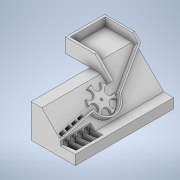
# Autodesk Inventor part: github
Saved by Autodesk Inventor 2020 (Build 240168000, 168)
## iProperties
Created: 2020-12-24
Part Number: github
Material: 一般
Document SubType Name: Modeling
Designer: Sugar
Density: 1 g/cm^3
Appearance: 預設
Author: Sugar
Autodesk Inventor part; units mm, degrees
ref_plane "YZ Plane" through (0, 0, 0) normal (1, 0, 0) x (0, 1, 0)
ref_plane "XZ Plane" through (0, 0, 0) normal (0, 1, 0) x (-1, 0, 0)
ref_plane "XY Plane" through (0, 0, 0) normal (0, 0, 1) x (1, 0, 0)
sketch "草圖2" plane through (0, 0, 0) normal (1, 0, 0) x (0, 1, 0)
  line L0 (0, 0) -> (300, 0)
  line L1 (300, 0) -> (300, 150)
  line L2 (300, 150) -> (150, 300)
  line L3 (150, 300) -> (100, 300)
  line L4 (100, 300) -> (100, 450)
  line L5 (100, 450) -> (0, 450)
  line L6 (0, 450) -> (0, 0)
  dimension "d0" = 300
  dimension "d1" = 450
  dimension "d2" = 150
  dimension "d3" = 150
  dimension "d4" = 100
  dimension "d5" = 50
  constraints: 14 end point, 4 perpendicular, 1 horizontal, 1 parallel
  measures "d0" distance of L0.start L0.end
  measures "d1" distance of L5.end L0.start
  measures "d2" distance of L0.end L1.end
  measures "d3" horizontal distance of L1.end L2.end
  measures "d4" distance of L4.end L5.end
  measures "d5" distance of L2.end L3.end
extrude "擠出1" add sketch "草圖2" along normal blind 600
sketch "草圖3" plane through (0, 150, 300) normal (0, 0.7071068, 0.7071068) x (1, 0, 0)
  line L0 (0, -212.132) -> (0, 106.066) projected
  line L1 (0, 0) -> (600, 0) projected
  line L2 (600, 106.066) -> (600, 318.1981) projected
  line L3 (0, 0) -> (350, 61.8718)
  line L4 (600, 106.066) -> (600, 121.066)
  line L5 (350, 76.8718) -> (0, 15)
  line L6 (0, 15) -> (0, 0)
  line L7 (350, 76.8718) -> (350, 61.8718)
  line L8 (600, 212.132) -> (600, 0) projected
  dimension "d11" = 15
  dimension "d31" = 250
  dimension "d32" = 15
  dimension "d33" = 14.771
  constraints: 10 end point, 2 parallel, 2 point on line, 1 collinear, 1 vertical
  measures "d11" distance of L2.start L4.end
  measures "d31" distance between parallel lines of L2 L7
  measures "d32" distance of L5.start L3.end
  measures "d33" distance between parallel lines of L3 L5
extrude "擠出3" add sketch "草圖3" along normal blind 60
sketch "草圖4" plane through (0, 300, 150) normal (0, 0.7071068, 0.7071068) x (1, 0, 0)
  circle A0 centre (225.2442, -146.9052) radius 10.25 construction
  circle A1 centre (179.5282, -153.9712) radius 11.25 construction
  circle A2 centre (98.546, -166.256) radius 13.25 construction
  circle A3 centre (46.5483, -174.4324) radius 14.25 construction
  line L0 (8.637, -195.6052) -> (251.57, -152.6603) construction
  line L1 (0, -197.132) -> (350, -135.2602) construction
  line L2 (14.7334, -165.5856) -> (63.97, -156.8817)
  line L3 (63.97, -156.8817) -> (68.9312, -184.9466)
  line L4 (14.7334, -165.5856) -> (19.6946, -193.6505)
  line L5 (88.6259, -181.465) -> (84.0128, -155.3696)
  line L6 (84.0128, -155.3696) -> (133.2494, -146.6658)
  line L7 (133.2494, -146.6658) -> (137.8625, -172.7612)
  line L8 (157.5571, -169.2796) -> (153.6404, -147.1231)
  line L9 (153.6404, -147.1231) -> (202.877, -138.4193)
  line L10 (202.877, -138.4193) -> (206.7937, -160.5757)
  line L11 (226.4883, -157.0942) -> (222.9198, -136.9072)
  line L12 (222.9198, -136.9072) -> (272.1563, -128.2033)
  line L13 (272.1563, -128.2033) -> (275.7249, -148.3903)
  line L14 (19.6946, -193.6505) -> (68.9312, -184.9466)
  line L15 (88.6259, -181.465) -> (137.8625, -172.7612)
  line L16 (157.5571, -169.2796) -> (206.7937, -160.5757)
  line L17 (226.4883, -157.0942) -> (275.7249, -148.3903)
  point P0 (0, -106.066)
  point P1 (600, -91.066)
  dimension "d17" = 20.5
  dimension "d18" = 22.5
  dimension "d19" = 26.5
  dimension "d20" = 28.5
  dimension "d21" = 50
  dimension "d22" = 50
  dimension "d23" = 50
  dimension "d24" = 50
  dimension "d25" = 20
  dimension "d26" = 20
  dimension "d27" = 20
  dimension "d28" = 20
  constraints: 34 end point, 10 perpendicular, 8 tangent, 4 centre point, 3 point on line, 2 collinear, 12 other
  measures "d17" diameter of A0
  measures "d18" diameter of A1
  measures "d19" diameter of A2
  measures "d20" diameter of A3
  measures "d21" distance between parallel lines of L4 L3
  measures "d22" distance between parallel lines of L7 L5
  measures "d23" distance between parallel lines of L10 L8
  measures "d24" distance between parallel lines of L13 L11
  measures "d25" distance between parallel lines of L10 L11
  measures "d26" distance between parallel lines of L7 L8
  measures "d27" distance between parallel lines of L3 L5
  measures "d28" distance from line of point (0, -197.132) L4
extrude "擠出4" cut sketch "草圖4" against normal blind 60
sketch "草圖5" plane through (350, 246.783, 288.0698) normal (-0.1740777, 0.6963106, -0.6963106) x (-0.9847319, -0.1230915, 0.1230915)
  line L0 (2.6112, -60) -> (358.0378, -60) projected
  line L1 (-8.4274, -60) -> (-8.4274, -120)
  line L2 (358.0378, -60) -> (2.6112, -60)
  line L3 (359.7659, -70) -> (-2.5175, -70)
  line L4 (125.4267, -120) -> (75.4267, -120) projected
  line L5 (75.4267, -120) -> (125.4267, -120) projected
  line L6 (195.4267, -120) -> (145.4267, -120) projected
  line L7 (145.4267, -120) -> (195.4267, -120) projected
  line L8 (265.4267, -120) -> (215.4267, -120) projected
  line L9 (215.4267, -120) -> (265.4267, -120) projected
  line L10 (335.4267, -120) -> (285.4267, -120) projected
  line L11 (285.4267, -120) -> (335.4267, -120) projected
  line L12 (75.4267, -120) -> (75.4267, -70)
  line L13 (75.4267, -120) -> (125.4267, -120)
  line L14 (125.4267, -120) -> (125.4267, -70)
  line L15 (145.4267, -70) -> (145.4267, -120)
  line L16 (145.4267, -120) -> (195.4267, -120)
  line L17 (195.4267, -120) -> (195.4267, -70)
  line L18 (215.4267, -70) -> (215.4267, -120)
  line L19 (215.4267, -120) -> (265.4267, -120)
  line L20 (265.4267, -120) -> (265.4267, -70)
  line L21 (285.4267, -70) -> (285.4267, -120)
  line L22 (285.4267, -120) -> (335.4267, -120)
  line L23 (335.4267, -120) -> (335.4267, -70)
  point P0 (339.5741, -378.1981)
  point P1 (75.4267, -120)
  point P2 (195.4267, -120)
  point P3 (215.4267, -120)
  point P4 (335.4267, -120)
  point P5 (285.4267, -120)
  dimension "d34" = 60
  dimension "d35" = 10
  constraints: 28 end point, 5 perpendicular, 3 horizontal, 3 parallel, 3 vertical, 1 collinear, 1 point on line, 11 other
  measures "d34" distance of L1.start L1.end
extrude "擠出7" cut sketch "草圖5" against normal blind 126 contours L14 L4 L12 L3
extrude "擠出8" cut sketch "草圖5" against normal blind 115 contours L17 L6 L15 L3
extrude "擠出9" cut sketch "草圖5" against normal blind 110 contours L20 L8 L18 L3
extrude "擠出10" cut sketch "草圖5" against normal blind 95 contours L23 L10 L21 L3
sketch "草圖10" plane through (0, 100, 450) normal (0, 1, 0) x (1, 0, 0)
  line L0 (33.694, 114.1421) -> (29.2117, 150) projected
  line L1 (79.987, 150) -> (84.4692, 114.1421) projected
  line L2 (104.7793, 114.1421) -> (100.2971, 150) projected
  line L3 (151.0723, 150) -> (155.5546, 114.1421) projected
  line L4 (175.8647, 114.1421) -> (171.3824, 150) projected
  line L5 (222.1577, 150) -> (226.6399, 114.1421) projected
  line L6 (246.5073, 117.6838) -> (242.4678, 150) projected
  line L7 (293.243, 150) -> (295.7439, 129.993) projected
  line L8 (0, 150) -> (600, 150) projected
  line L9 (24.1728, 150) -> (39.1728, 30)
  line L10 (39.1728, 30) -> (100.0259, 30)
  line L11 (100.0259, 30) -> (85.0259, 150)
  line L12 (24.1728, 150) -> (85.0259, 150)
  line L13 (95.2582, 150) -> (110.2582, 30)
  line L14 (110.2582, 30) -> (171.1112, 30)
  line L15 (171.1112, 30) -> (156.1112, 150)
  line L16 (95.2582, 150) -> (156.1112, 150)
  line L17 (166.3435, 150) -> (181.3435, 30)
  line L18 (181.3435, 30) -> (242.1966, 30)
  line L19 (242.1966, 30) -> (227.1966, 150)
  line L20 (166.3435, 150) -> (227.1966, 150)
  line L21 (237.4288, 150) -> (252.4288, 30)
  line L22 (252.4288, 30) -> (313.2819, 30)
  line L23 (313.2819, 30) -> (298.2819, 150)
  line L24 (237.4288, 150) -> (298.2819, 150)
  line L25 (0, 0) -> (600, 0) projected
  point P0 (0, 450)
  point P1 (225.9422, 119.7233)
  point P2 (294.8735, 136.9561)
  point P3 (245.6369, 124.647)
  point P4 (225.9422, 119.7233)
  point P5 (104.7793, 114.1421)
  point P6 (155.5546, 114.1421)
  point P7 (33.694, 114.1421)
  point P8 (84.4692, 114.1421)
  point P9 (24.1728, 150)
  dimension "d17" = 20.5
  dimension "d18" = 22.5
  dimension "d19" = 26.5
  dimension "d20" = 28.5
  dimension "d21" = 50
  dimension "d22" = 50
  dimension "d23" = 50
  dimension "d24" = 50
  dimension "d25" = 20
  dimension "d26" = 20
  dimension "d27" = 20
  dimension "d28" = 20
  dimension "d39" = 30
  dimension "d40" = 30
  dimension "d41" = 30
  dimension "d42" = 30
  dimension "d45" = 5
  dimension "d46" = 5
  dimension "d47" = 5
  dimension "d48" = 5
  dimension "d49" = 5
  dimension "d50" = 5
  dimension "d51" = 5
  dimension "d52" = 5
  constraints: 32 end point, 13 parallel, 4 point on line
  measures "d39" distance between parallel lines of L25 L10
  measures "d40" distance between parallel lines of L25 L14
  measures "d41" distance between parallel lines of L25 L18
  measures "d42" distance between parallel lines of L25 L22
  measures "d45" distance between parallel lines of L11 L1
  measures "d46" distance between parallel lines of L0 L9
  measures "d47" distance between parallel lines of L2 L13
  measures "d48" distance between parallel lines of L15 L3
  measures "d49" distance between parallel lines of L4 L17
  measures "d50" distance between parallel lines of L5 L19
  measures "d51" distance between parallel lines of L7 L23
  measures "d52" distance between parallel lines of L6 L21
extrude "擠出6" cut sketch "草圖10" against normal blind 65
sketch "草圖11" plane through (0, 300, 150) normal (0, 0.7071068, 0.7071068) x (1, 0, 0)
  circle A0 centre (477.6204, -106.066) radius 127.6204
  line L0 (600, 0) -> (600, -212.132) projected
  line L1 (350, -135.2602) -> (350, -150.2602) projected
  point P0 (0, -106.066)
  point P1 (600, -106.066)
  point P2 (600, -142.2624)
  point P3 (600, -69.8697)
  constraints: 1 centre point, 1 horizontal alignment, 1 midpoint, 1 tangent
extrude "擠出11" add sketch "草圖11" along normal blind 20
sketch "草圖12" plane through (0, 314.1421, 164.1421) normal (0, 0.7071068, 0.7071068) x (1, 0, 0)
  circle A0 centre (477.6204, -106.066) radius 127.6204 projected
  circle A1 centre (477.6204, -106.066) radius 10
  circle A2 centre (402.5525, -36.0873) radius 40
  line L0 (0, -106.066) -> (600, -106.066) projected
  circle A3 centre (379.4831, -136.0873) radius 40
  circle A4 centre (454.551, -206.066) radius 40
  circle A5 centre (552.6882, -176.0447) radius 40
  circle A6 centre (575.7576, -76.0447) radius 40
  circle A7 centre (500.6897, -6.066) radius 40
  line L1 (500.6897, -6.066) -> (477.6204, -106.066) construction
  line L2 (364.1482, -99.1436) -> (350.0043, -105.0145)
  line L3 (394.818, -173.0311) -> (374.6185, -181.4157)
  line L4 (364.1482, -99.1436) -> (394.818, -173.0311) construction
  line L5 (415.5747, -197.0744) -> (493.5272, -215.0576) construction
  line L6 (454.551, -206.066) -> (477.6204, -106.066) construction
  line L7 (415.5747, -197.0744) -> (411.4018, -215.1626)
  line L8 (493.5272, -215.0576) -> (489.3544, -233.1458)
  line L9 (552.6882, -176.0447) -> (477.6204, -106.066) construction
  line L10 (525.4131, -205.3034) -> (579.9633, -146.786) construction
  line L11 (402.5525, -36.0873) -> (477.6204, -106.066) construction
  line L12 (379.4831, -136.0873) -> (477.6204, -106.066) construction
  line L13 (575.7576, -76.0447) -> (477.6204, -106.066) construction
  line L14 (525.4131, -205.3034) -> (538.9915, -217.9612)
  line L15 (579.9633, -146.786) -> (593.5417, -159.4439)
  line L16 (564.0564, -37.7944) -> (587.4588, -114.295) construction
  line L17 (564.0564, -37.7944) -> (581.8076, -32.3641)
  line L18 (587.4588, -114.295) -> (605.21, -108.8647)
  line L19 (461.7135, 2.9256) -> (465.8863, 21.0137)
  line L20 (500.6897, -6.066) -> (539.666, -15.0576) construction
  line L21 (500.6897, -6.066) -> (461.7135, 2.9256) construction
  line L22 (539.666, -15.0576) -> (543.8389, 3.0306)
  line L23 (375.2774, -65.346) -> (429.8276, -6.8287) construction
  line L24 (375.2774, -65.346) -> (361.699, -52.6881)
  line L25 (429.8276, -6.8287) -> (416.2492, 5.8292)
  point P0 (600, -69.8697)
  point P1 (600, -142.2624)
  point P2 (471.6228, 21.4133)
  point P3 (538.8571, 5.9028)
  point P4 (605.2066, -103.1142)
  point P5 (585.0219, -37.1323)
  point P6 (591.0195, -164.6117)
  point P7 (543.9698, -215.083)
  point P8 (416.3836, -218.0348)
  point P9 (483.6179, -233.5454)
  point P10 (350.0341, -109.0178)
  point P11 (370.2188, -174.9997)
  point P12 (411.2709, 2.951)
  point P13 (364.2212, -47.5203)
  dimension "d63" = 20
  dimension "d64" = 80
  dimension "d67" = 360
  dimension "d69" = 100
  constraints: 50 end point, 17 perpendicular, 17 point on circle, 7 centre point, 5 midpoint, 5 tangent, 1 coincident, 1 collinear, 26 other
  measures "d63" diameter of A1
  measures "d64" diameter of A2
  measures "d69" vertical distance of L1.start L1.end
extrude "擠出12" cut sketch "草圖12" against normal blind 20 contours A0 A6 L17 | L22 A7 A0 | A0 A6 | A7 A0 | A0 L18 A6 | A7 L19 A0 | L0 A1 | A1 L0 | L25 A2 A0 | A0 A5 L15 | A3 A0 L0 | L0 A3 | A2 A0 | A0 A5 | A3 A0 L0 | L0 A0 L2 A3 | A2 L24 A0 | A0 L14 A5 | L3 A0 A3 | A0 A4 L8 | L7 A4 A0 | A0 A4 picked at (578.5347, -74.0136) picked at (502.7839, -3.1882) picked at (399.3169, -34.7769) picked at (556.034, -177.2583) picked at (455.0481, -209.5281)
sketch "草圖13" plane through (0, 314.1421, 164.1421) normal (0, 0.7071068, 0.7071068) x (1, 0, 0)
  arc A0 (394.818, -173.0311) -> (364.1482, -99.1436) centre (379.4831, -136.0873) ccw projected
  arc A1 (593.5417, -159.4439) -> (605.21, -108.8647) centre (477.6204, -106.066) ccw projected
  arc A2 (493.5272, -215.0576) -> (415.5747, -197.0744) centre (454.551, -206.066) ccw projected
  arc A3 (581.8076, -32.3641) -> (543.8389, 3.0306) centre (477.6204, -106.066) ccw projected
  arc A4 (579.9633, -146.786) -> (525.4131, -205.3034) centre (552.6882, -176.0447) ccw projected
  arc A5 (465.8863, 21.0137) -> (416.2492, 5.8292) centre (477.6204, -106.066) ccw projected
  arc A6 (564.0564, -37.7944) -> (587.4588, -114.295) centre (575.7576, -76.0447) ccw projected
  arc A7 (361.699, -52.6881) -> (350.0043, -105.0145) centre (477.6204, -106.066) ccw projected
  arc A8 (461.7135, 2.9256) -> (539.666, -15.0576) centre (500.6897, -6.066) ccw projected
  arc A9 (374.6185, -181.4157) -> (411.4018, -215.1626) centre (477.6204, -106.066) ccw projected
  arc A10 (375.2774, -65.346) -> (429.8276, -6.8287) centre (402.5525, -36.0873) ccw projected
  arc A11 (489.3544, -233.1458) -> (538.9915, -217.9612) centre (477.6204, -106.066) ccw projected
  circle A12 centre (477.6204, -106.066) radius 10 projected
  line L0 (0, -212.132) -> (350, -150.2602) projected
  arc A13 (350, -150.2602) -> (610.3108, -131.2321) centre (477.6204, -106.066) ccw
  arc A14 (335.0608, -152.9011) -> (625.5508, -131.2321) centre (477.6204, -106.066) ccw
  line L1 (350, -135.2602) -> (350, -150.2602) projected
  line L2 (350, -150.2602) -> (335.0608, -152.9011)
  line L3 (610.3108, -131.2321) -> (625.5508, -131.2321)
  line L4 (394.818, -173.0311) -> (374.6185, -181.4157) projected
  line L5 (411.4018, -215.1626) -> (415.5747, -197.0744) projected
  line L6 (493.5272, -215.0576) -> (489.3544, -233.1458) projected
  line L7 (538.9915, -217.9612) -> (525.4131, -205.3034) projected
  line L8 (579.9633, -146.786) -> (593.5417, -159.4439) projected
  line L9 (605.21, -108.8647) -> (587.4588, -114.295) projected
  line L10 (564.0564, -37.7944) -> (581.8076, -32.3641) projected
  line L11 (543.8389, 3.0306) -> (539.666, -15.0576) projected
  line L12 (461.7135, 2.9256) -> (465.8863, 21.0137) projected
  line L13 (416.2492, 5.8292) -> (429.8276, -6.8287) projected
  line L14 (375.2774, -65.346) -> (361.699, -52.6881) projected
  line L15 (350.0043, -105.0145) -> (364.1482, -99.1436) projected
  point P0 (0, -106.066)
  dimension "d72" = 15
  constraints: 5 end point, 4 point on circle, 2 centre point, 2 coincident, 1 horizontal, 1 point on line
  measures "d72" radial gap between concentric circles of A14 A13
extrude "擠出13" add sketch "草圖13" along normal mid plane 80 contours L0 A13 L3 A14
sketch "草圖14" plane through (0, 150, 300) normal (0, 0.7071068, 0.7071068) x (1, 0, 0)
  line L0 (600, -212.132) -> (600, 106.066) projected
  line L1 (600, 8.2369) -> (304.413, 8.2369)
  line L2 (304.413, 8.2369) -> (304.413, -70.0383)
  line L3 (304.413, -70.0383) -> (600, -70.0383)
  line L4 (600, -70.0383) -> (600, 8.2369)
  arc A0 (396.2317, -20) -> (559.009, -20) centre (477.6204, 106.066) ccw projected
  line L5 (298.2819, -35.3553) -> (313.2819, -120.2082) projected
  point P0 (0, 106.066)
  point P1 (600, -70.0383)
  constraints: 8 end point, 2 parallel, 2 point on line, 1 horizontal, 1 perpendicular
extrude "擠出14" add sketch "草圖14" against normal blind 85
sketch "草圖15" plane through (0, 300, 150) normal (0, 0.7071068, 0.7071068) x (1, 0, 0)
  line L0 (600, -106.066) -> (600, 106.066) projected
  line L1 (0, 0) -> (600, 0)
  line L2 (600, 0) -> (600, 56.5167)
  line L3 (600, 56.5167) -> (0, 56.5167)
  line L4 (0, 56.5167) -> (0, 0)
  point P0 (0, -106.066)
  point P1 (600, 0)
  constraints: 8 end point, 2 parallel, 1 horizontal, 1 perpendicular, 1 point on line
extrude "擠出15" add sketch "草圖15" against normal blind 80
sketch "草圖17" plane through (600, 0, 0) normal (1, 0, 0) x (0, 0, -1)
  line L0 (-228.1059, 221.8941) -> (-110.0367, 339.9633) projected
  line L1 (-228.1059, 221.8941) -> (-250.5947, 199.4053) projected
  line L2 (-250.5947, 199.4053) -> (-265.3937, 184.6063) projected
  line L3 (-265.3937, 184.6063) -> (-251.2516, 170.4642) projected
  line L4 (-251.2516, 170.4642) -> (-272.2581, 149.4576) projected
  line L5 (-272.2581, 149.4576) -> (-286.4002, 163.5998) projected
  line L6 (-286.4002, 163.5998) -> (-349.5246, 100.4754) projected
  line L7 (-349.5246, 100.4754) -> (-349.0491, 100) projected
  line L8 (-349.0491, 100) -> (-450, 100) projected
  line L9 (-450, 100) -> (-450, 0) projected
  line L10 (-450, 0) -> (0, 0) projected
  line L11 (0, 0) -> (0, 300) projected
  line L12 (0, 300) -> (-70.0734, 300) projected
  line L13 (-110.0367, 339.9633) -> (-70.0734, 300) projected
  line L14 (0, 300) -> (-70.0734, 300) projected
  line L15 (-450, 0) -> (0, 0) projected
  line L16 (0, 300) -> (-150, 300)
  line L17 (-150, 300) -> (-150, 0)
  line L18 (-150, 0) -> (0, 0)
  line L19 (0, 0) -> (0, 300)
  line L20 (-286.4002, 163.5998) -> (-286.4002, 0)
  line L21 (-150, 300) -> (-286.4002, 163.5998)
  line L22 (-295.1714, 154.8286) -> (-246.1981, 203.8019) projected
  line L23 (-286.4002, 163.5998) -> (-349.5246, 100.4754)
  line L24 (-267.4264, 182.5736) -> (-302.0687, 147.9313) projected
  line L25 (-350, 100) -> (-450, 100)
  line L26 (-450, 100) -> (-450, 0)
  line L27 (-450, 0) -> (-286.4002, 0)
  point P0 (-150, 0)
  point P1 (-70.0734, 300)
  point P2 (-253.7934, 196.2066)
  point P3 (-286.4002, 0)
  point P4 (-289.3527, 160.6473)
  constraints: 20 end point, 4 point on line, 3 collinear, 2 horizontal, 2 parallel, 2 perpendicular, 1 vertical
extrude "擠出16" add sketch "草圖17" along normal blind 400 contours L0 L17 L10 L20 L5 L4 L3 L2 L1 | L16 L12 L11 L10 L17 | L3 L4 L5 L21
sketch "草圖18" plane through (0, 339.9633, 110.0367) normal (0, 0.7071068, 0.7071068) x (1, 0, 0)
  line L0 (600, -56.5167) -> (600, 0) projected
  line L1 (600, 0) -> (0, 0) projected
  line L2 (0, 0) -> (0, -253.6487) projected
  line L3 (0, -253.6487) -> (19.6946, -250.1671) projected
  line L4 (19.6946, -250.1671) -> (14.7334, -222.1023) projected
  line L5 (14.7334, -222.1023) -> (63.97, -213.3984) projected
  line L6 (63.97, -213.3984) -> (68.9312, -241.4633) projected
  line L7 (68.9312, -241.4633) -> (88.6259, -237.9817) projected
  line L8 (88.6259, -237.9817) -> (84.0128, -211.8863) projected
  line L9 (84.0128, -211.8863) -> (133.2494, -203.1824) projected
  line L10 (133.2494, -203.1824) -> (137.8625, -229.2778) projected
  line L11 (137.8625, -229.2778) -> (157.5571, -225.7963) projected
  line L12 (157.5571, -225.7963) -> (153.6404, -203.6398) projected
  line L13 (153.6404, -203.6398) -> (202.877, -194.9359) projected
  line L14 (202.877, -194.9359) -> (206.7937, -217.0924) projected
  line L15 (206.7937, -217.0924) -> (226.4883, -213.6108) projected
  line L16 (226.4883, -213.6108) -> (222.9198, -193.4238) projected
  line L17 (222.9198, -193.4238) -> (272.1563, -184.7199) projected
  line L18 (272.1563, -184.7199) -> (275.7249, -204.907) projected
  line L19 (275.7249, -204.907) -> (350, -191.7769) projected
  line L20 (350, -191.7769) -> (350, -206.7769) projected
  arc A0 (350, -206.7769) -> (610.3108, -187.7487) centre (477.6204, -162.5827) ccw projected
  line L21 (625.5508, -187.7487) -> (610.3108, -187.7487) projected
  arc A1 (600, -249.4157) -> (625.5508, -187.7487) centre (477.6204, -162.5827) ccw projected
  line L22 (600, -249.4157) -> (1000, -249.4157) projected
  line L23 (1000, -56.5167) -> (1000, -249.4157) projected
  line L24 (600, -56.5167) -> (1000, -56.5167) projected
  line L25 (587.4588, -170.8116) -> (605.21, -165.3813) projected
  arc A2 (593.5417, -215.9606) -> (605.21, -165.3813) centre (477.6204, -162.5827) ccw projected
  line L26 (579.9633, -203.3027) -> (593.5417, -215.9606) projected
  arc A3 (579.9633, -203.3027) -> (525.4131, -261.82) centre (552.6882, -232.5614) ccw projected
  line L27 (525.4131, -261.82) -> (538.9915, -274.4779) projected
  arc A4 (489.3544, -289.6624) -> (538.9915, -274.4779) centre (477.6204, -162.5827) ccw projected
  line L28 (489.3544, -289.6624) -> (493.5272, -271.5743) projected
  arc A5 (493.5272, -271.5743) -> (415.5747, -253.5911) centre (454.551, -262.5827) ccw projected
  line L29 (415.5747, -253.5911) -> (411.4018, -271.6792) projected
  arc A6 (374.6185, -237.9323) -> (411.4018, -271.6792) centre (477.6204, -162.5827) ccw projected
  line L30 (394.818, -229.5477) -> (374.6185, -237.9323) projected
  arc A7 (394.818, -229.5477) -> (364.1482, -155.6603) centre (379.4831, -192.604) ccw projected
  line L31 (350.0043, -161.5312) -> (364.1482, -155.6603) projected
  arc A8 (361.699, -109.2048) -> (350.0043, -161.5312) centre (477.6204, -162.5827) ccw projected
  line L32 (375.2774, -121.8627) -> (361.699, -109.2048) projected
  arc A9 (375.2774, -121.8627) -> (429.8276, -63.3453) centre (402.5525, -92.604) ccw projected
  line L33 (429.8276, -63.3453) -> (416.2492, -50.6875) projected
  arc A10 (465.8863, -35.5029) -> (416.2492, -50.6875) centre (477.6204, -162.5827) ccw projected
  line L34 (465.8863, -35.5029) -> (461.7135, -53.5911) projected
  arc A11 (461.7135, -53.5911) -> (539.666, -71.5743) centre (500.6897, -62.5827) ccw projected
  line L35 (539.666, -71.5743) -> (543.8389, -53.4861) projected
  arc A12 (581.8076, -88.8808) -> (543.8389, -53.4861) centre (477.6204, -162.5827) ccw projected
  line L36 (564.0564, -94.3111) -> (581.8076, -88.8808) projected
  arc A13 (564.0564, -94.3111) -> (587.4588, -170.8116) centre (575.7576, -132.5614) ccw projected
  line L37 (600, -56.5167) -> (1000, -56.5167) projected
  line L38 (600, -56.5167) -> (1000, -56.5167)
  line L39 (1000, -56.5167) -> (1000, 143.4833)
  line L40 (1000, 143.4833) -> (600, 143.4833)
  line L41 (600, 143.4833) -> (600, -56.5167)
  point P0 (0, -162.5827)
  dimension "d81" = 200
  constraints: 8 end point, 2 parallel, 1 horizontal, 1 perpendicular
  measures "d81" distance between parallel lines of L24 L40
extrude "擠出17" add sketch "草圖18" against normal blind 200 contours L0 L41 L40 L39 L24
sketch "草圖19" plane through (600, 163.5998, 286.4002) normal (0, 0.7071068, 0.7071068) x (1, 0, 0)
  line L0 (0, 249.4157) -> (-600, 249.4157) projected
  line L1 (-600, 249.4157) -> (-600, -4.233) projected
  line L2 (-600, -4.233) -> (-580.3054, -0.7514) projected
  line L3 (-580.3054, -0.7514) -> (-585.2666, 27.3134) projected
  line L4 (-585.2666, 27.3134) -> (-536.03, 36.0173) projected
  line L5 (-536.03, 36.0173) -> (-531.0688, 7.9525) projected
  line L6 (-531.0688, 7.9525) -> (-511.3741, 11.434) projected
  line L7 (-511.3741, 11.434) -> (-515.9872, 37.5294) projected
  line L8 (-515.9872, 37.5294) -> (-466.7506, 46.2333) projected
  line L9 (-466.7506, 46.2333) -> (-462.1375, 20.1379) projected
  line L10 (-462.1375, 20.1379) -> (-442.4429, 23.6194) projected
  line L11 (-442.4429, 23.6194) -> (-446.3596, 45.7759) projected
  line L12 (-446.3596, 45.7759) -> (-397.123, 54.4798) projected
  line L13 (-397.123, 54.4798) -> (-393.2063, 32.3233) projected
  line L14 (-393.2063, 32.3233) -> (-373.5117, 35.8049) projected
  line L15 (-373.5117, 35.8049) -> (-377.0802, 55.9919) projected
  line L16 (-377.0802, 55.9919) -> (-327.8437, 64.6958) projected
  line L17 (-327.8437, 64.6958) -> (-324.2751, 44.5088) projected
  line L18 (-324.2751, 44.5088) -> (-250, 57.6389) projected
  line L19 (-250, 57.6389) -> (-250, 42.6389) projected
  arc A0 (-250, 42.6389) -> (10.3108, 61.667) centre (-122.3796, 86.833) ccw projected
  line L20 (25.5508, 61.667) -> (10.3108, 61.667) projected
  arc A1 (0, 0) -> (25.5508, 61.667) centre (-122.3796, 86.833) ccw projected
  line L21 (0, 0) -> (400, 0) projected
  line L22 (400, 0) -> (400, 392.899) projected
  line L23 (400, 392.899) -> (0, 392.899) projected
  line L24 (0, 392.899) -> (0, 249.4157) projected
  line L25 (-12.5412, 78.6041) -> (5.21, 84.0344) projected
  arc A2 (-6.4583, 33.4551) -> (5.21, 84.0344) centre (-122.3796, 86.833) ccw projected
  line L26 (-20.0367, 46.113) -> (-6.4583, 33.4551) projected
  arc A3 (-20.0367, 46.113) -> (-74.5869, -12.4043) centre (-47.3118, 16.8543) ccw projected
  line L27 (-74.5869, -12.4043) -> (-61.0085, -25.0622) projected
  arc A4 (-110.6456, -40.2467) -> (-61.0085, -25.0622) centre (-122.3796, 86.833) ccw projected
  line L28 (-110.6456, -40.2467) -> (-106.4728, -22.1586) projected
  arc A5 (-106.4728, -22.1586) -> (-184.4253, -4.1754) centre (-145.449, -13.167) ccw projected
  line L29 (-184.4253, -4.1754) -> (-188.5982, -22.2635) projected
  arc A6 (-225.3815, 11.4834) -> (-188.5982, -22.2635) centre (-122.3796, 86.833) ccw projected
  line L30 (-205.182, 19.868) -> (-225.3815, 11.4834) projected
  arc A7 (-205.182, 19.868) -> (-235.8518, 93.7555) centre (-220.5169, 56.8117) ccw projected
  line L31 (-249.9957, 87.8845) -> (-235.8518, 93.7555) projected
  arc A8 (-238.301, 140.2109) -> (-249.9957, 87.8845) centre (-122.3796, 86.833) ccw projected
  line L32 (-224.7226, 127.5531) -> (-238.301, 140.2109) projected
  arc A9 (-224.7226, 127.5531) -> (-170.1724, 186.0704) centre (-197.4475, 156.8117) ccw projected
  line L33 (-170.1724, 186.0704) -> (-183.7508, 198.7282) projected
  arc A10 (-134.1137, 213.9128) -> (-183.7508, 198.7282) centre (-122.3796, 86.833) ccw projected
  line L34 (-134.1137, 213.9128) -> (-138.2865, 195.8246) projected
  arc A11 (-138.2865, 195.8246) -> (-60.334, 177.8414) centre (-99.3103, 186.833) ccw projected
  line L35 (-60.334, 177.8414) -> (-56.1611, 195.9296) projected
  arc A12 (-18.1924, 160.5349) -> (-56.1611, 195.9296) centre (-122.3796, 86.833) ccw projected
  line L36 (-35.9436, 155.1046) -> (-18.1924, 160.5349) projected
  arc A13 (-35.9436, 155.1046) -> (-12.5412, 78.6041) centre (-24.2424, 116.8543) ccw projected
  line L37 (25.5508, 61.667) -> (10.3108, 61.667) projected
  line L38 (0, 392.899) -> (25, 392.899)
  line L39 (25, 392.899) -> (25, 161.667)
  line L40 (25, 161.667) -> (0, 161.667)
  line L41 (0, 161.667) -> (0, 392.899)
  line L42 (40.3108, 61.667) -> (400, 301.4598)
  line L43 (10.3108, 61.667) -> (400, 321.4598)
  line L44 (400, 0) -> (400, 392.899) projected
  line L45 (400, 321.4598) -> (400, 301.4598)
  line L46 (400, 321.4598) -> (400, 392.899)
  line L47 (400, 392.899) -> (0, 392.899) projected
  line L48 (400, 392.899) -> (380, 392.899)
  line L49 (380, 392.899) -> (380, 308.1265)
  line L50 (10.3108, 61.667) -> (40.3108, 61.667)
  line L51 (40.3108, 61.667) -> (22.0498, 49.493)
  point P0 (-600, 86.833)
  point P1 (25, 392.899)
  point P2 (25.5508, 61.667)
  point P3 (380, 392.899)
  point P4 (23.1411, 50.2205)
  point P5 (25.5508, 61.667)
  dimension "d84" = 20
  dimension "d85" = 25
  dimension "d86" = 100
  dimension "d87" = 30
  dimension "d88" = 20
  constraints: 24 end point, 4 point on line, 3 parallel, 2 collinear, 2 horizontal, 2 perpendicular
  measures "d84" distance between parallel lines of L22 L49
  measures "d85" distance between parallel lines of L24 L39
  measures "d86" distance between parallel lines of L20 L40
  measures "d87" distance of L20.end L42.start
  measures "d88" distance of L42.end L43.end
extrude "擠出18" add sketch "草圖19" along normal up to surface (60 mm away) contours L24 L23 L39 L40 L41 | L23 L22 L43 L49 | L43 L22 L42 L50 L20 | L50 L51 A1
sketch "草圖20" plane through (600, 0, 0) normal (1, 0, 0) x (0, 0, -1)
  line L0 (-286.4002, 0) -> (-286.4002, 163.5998) projected
  line L1 (-286.4002, 163.5998) -> (-349.5246, 100.4754) projected
  line L2 (-349.5246, 100.4754) -> (-349.0491, 100) projected
  line L3 (-349.0491, 100) -> (-450, 100) projected
  line L4 (-450, 100) -> (-450, 0) projected
  line L5 (-450, 0) -> (-286.4002, 0) projected
  line L6 (-300, 100) -> (-450, 100) projected
  line L7 (-349.0491, 100) -> (-450, 100)
  line L8 (-450, 100) -> (-450, 0)
  line L9 (-450, 0) -> (-286.4002, 0) projected
  line L10 (-450, 0) -> (-286.4002, 0)
  line L11 (-286.4002, 0) -> (-286.4002, 163.5998)
  point P0 (0, 0)
  constraints: 8 end point, 2 perpendicular, 1 horizontal, 1 parallel, 1 point on line
extrude "擠出19" add sketch "草圖20" along normal blind 400
sketch "草圖21" plane through (0, 0, 0) normal (-1, 0, 0) x (0, 0, 1)
  line L0 (0, 300) -> (0, 167.1573) projected
  line L1 (70.0734, 300) -> (0, 300) projected
  line L2 (110.0367, 339.9633) -> (70.0734, 300) projected
  line L3 (172.0844, 277.9156) -> (110.0367, 339.9633) projected
  line L4 (172.0844, 277.9156) -> (214.5108, 320.342) projected
  line L5 (214.5108, 320.342) -> (51.0051, 483.8478) projected
  line L6 (51.0051, 483.8478) -> (-132.8427, 300) projected
  line L7 (0, 167.1573) -> (-132.8427, 300) projected
  line L8 (0, 167.1573) -> (0, 432.8427)
  line L9 (-132.8427, 300) -> (0, 167.1573) projected
  line L10 (-132.8427, 300) -> (0, 432.8427)
  line L11 (-132.8427, 300) -> (51.0051, 483.8478) projected
  line L12 (-132.8427, 300) -> (0, 167.1573)
  point P0 (0, 0)
  constraints: 6 end point, 2 collinear, 1 point on line, 1 vertical
extrude "擠出20" cut sketch "草圖21" against normal through all contours L0 L7 L6 L8
sketch "草圖22" plane through (0, 0, 0) normal (-1, 0, 0) x (0, 0, 1)
  line L0 (0, 300) -> (70.0734, 300) projected
  line L1 (0, 0) -> (0, 300) projected
  line L2 (450, 0) -> (0, 0) projected
  line L3 (450, 100) -> (450, 0) projected
  line L4 (300, 100) -> (450, 100) projected
  line L5 (300, 150) -> (300, 100) projected
  line L6 (300, 150) -> (342.4264, 192.4264) projected
  line L7 (331.8198, 203.033) -> (342.4264, 192.4264) projected
  line L8 (289.3934, 160.6066) -> (331.8198, 203.033) projected
  line L9 (110.0367, 339.9633) -> (289.3934, 160.6066) projected
  line L10 (110.0367, 339.9633) -> (70.0734, 300) projected
  line L11 (110.0367, 339.9633) -> (0, 339.9633)
  line L12 (0, 300) -> (70.0734, 300) projected
  line L13 (110.0367, 339.9633) -> (70.0734, 300)
  line L14 (70.0734, 300) -> (0, 300)
  line L15 (0, 300) -> (0, 339.9633)
  constraints: 8 end point, 1 collinear, 1 horizontal, 1 perpendicular
extrude "擠出21" add sketch "草圖22" against normal blind 600 contours L15 L11 L10 L0
sketch "草圖25" plane through (1000, 0, 0) normal (0, 0, -1) x (-1, 0, 0)
  line L0 (0, 432.8427) -> (400, 432.8427) projected
  line L1 (400, 483.8478) -> (400, 432.8427) projected
  line L2 (400, 483.8478) -> (375, 483.8478) projected
  line L3 (375, 441.4214) -> (375, 483.8478) projected
  line L4 (20, 441.4214) -> (375, 441.4214) projected
  line L5 (20, 441.4214) -> (20, 483.8478) projected
  line L6 (20, 483.8478) -> (0, 483.8478) projected
  line L7 (0, 432.8427) -> (0, 483.8478) projected
  line L8 (0, 0) -> (0, 432.8427) projected
  line L9 (1000, 0) -> (0, 0) projected
  line L10 (1000, 0) -> (1000, 339.9633) projected
  line L11 (1000, 339.9633) -> (400, 339.9633) projected
  line L12 (400, 432.8427) -> (400, 339.9633) projected
  line L13 (0, 432.8427) -> (400, 432.8427) projected
  line L14 (400, 483.8478) -> (375, 483.8478) projected
  line L15 (0, 0) -> (0, 432.8427) projected
  line L16 (400, 483.8478) -> (0, 483.8478)
  line L17 (0, 483.8478) -> (0, 339.9633)
  line L18 (0, 339.9633) -> (400, 339.9633)
  line L19 (400, 339.9633) -> (400, 483.8478)
  constraints: 8 end point, 2 parallel, 1 collinear, 1 horizontal, 1 perpendicular, 1 point on line
extrude "擠出24" add sketch "草圖25" along normal blind 250 and the other way blind 50 contours L7 L6 L5 L4 L3 L2 L1 L0 | L0 L12 L18 L8 | L16 L3 L4 L5
sketch "草圖26" plane through (1000, 0, 50) normal (0, 0, 1) x (1, 0, 0)
  line L0 (-375, 482.8427) -> (-400, 482.8427) projected
  line L1 (-375, 400) -> (-375, 482.8427) projected
  line L2 (-20, 400) -> (-375, 400) projected
  line L3 (-20, 482.8427) -> (-20, 400) projected
  line L4 (0, 482.8427) -> (-20, 482.8427) projected
  line L5 (0, 482.8427) -> (0, 483.8478) projected
  line L6 (0, 483.8478) -> (-400, 483.8478) projected
  line L7 (-400, 483.8478) -> (-400, 482.8427) projected
  line L8 (-20, 423.9045) -> (-20, 483.8478) projected
  line L9 (-375, 400) -> (-375, 277.9156) projected
  line L10 (-20, 483.8478) -> (-375, 483.8478)
  line L11 (-375, 483.8478) -> (-375, 400)
  line L12 (-375, 400) -> (-20, 400)
  line L13 (-20, 400) -> (-20, 483.8478)
  point P0 (-1000, 0)
  constraints: 8 end point, 2 parallel, 1 horizontal, 1 perpendicular
extrude "擠出25" cut sketch "草圖26" against normal blind 275 contours L11 L6 L8 L3 L2 L1
sketch "草圖27" plane through (1000, 0, 50) normal (0, 0, 1) x (1, 0, 0)
  line L0 (-20, 483.8478) -> (-20, 482.8427) projected
  line L1 (0, 482.8427) -> (-20, 482.8427) projected
  line L2 (0, 482.8427) -> (0, 483.8478) projected
  line L3 (0, 483.8478) -> (-20, 483.8478) projected
  line L4 (-375, 482.8427) -> (-375, 483.8478) projected
  line L5 (-375, 483.8478) -> (-400, 483.8478) projected
  line L6 (-400, 483.8478) -> (-400, 482.8427) projected
  line L7 (-375, 482.8427) -> (-400, 482.8427) projected
  line L8 (0, 483.758) -> (-20, 483.758)
  line L9 (-20, 483.758) -> (-20, 482.8427)
  line L10 (-20, 482.8427) -> (0, 482.8427)
  line L11 (0, 482.8427) -> (0, 483.758)
  line L12 (-375, 483.8478) -> (-400, 483.8478)
  line L13 (-400, 483.8478) -> (-400, 482.8427)
  line L14 (-400, 482.8427) -> (-375, 482.8427)
  line L15 (-375, 482.8427) -> (-375, 483.8478)
  point P0 (-1000, 0)
  constraints: 16 end point, 4 parallel, 2 horizontal, 2 perpendicular, 1 point on line
extrude "擠出26" add sketch "草圖27" along normal blind 1
